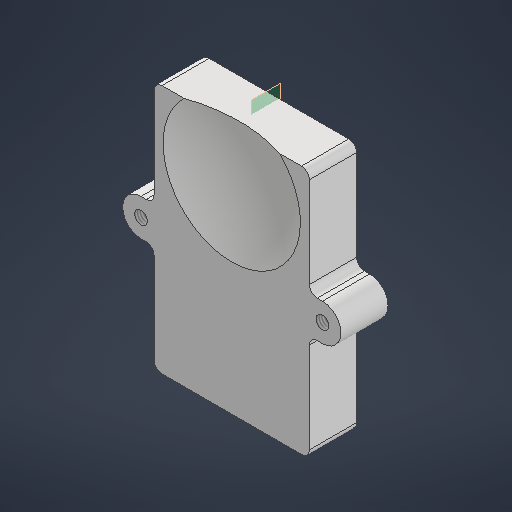
# Autodesk Inventor part: SphereMount
Saved by Autodesk Inventor 2025.1 (Build 291241020, 241B)
## iProperties
Created: 2024-09-20
Part Number: SphereMount
Material: Generic
Document SubType Name: Modeling
Designer: Sora
Density: 1 g/cm^3
Appearance: Default
Author: Sora
Autodesk Inventor part; units mm, degrees
ref_plane "YZ Plane" through (0, 0, 0) normal (1, 0, 0) x (0, 1, 0)
ref_plane "XZ Plane" through (0, 0, 0) normal (0, 1, 0) x (-1, 0, 0)
ref_plane "XY Plane" through (0, 0, 0) normal (0, 0, 1) x (1, 0, 0)
sketch "Sketch1" plane through (0, 0, 0) normal (0, 0, 1) x (1, 0, 0)
  arc A0 (-3.85, 3.05) -> (-3.85, -3.95) centre (-3.85, -0.45) ccw projected
  arc A1 (-1.4191, -5) -> (-2.85, -3.95) centre (-2.85, -5.45) ccw projected
  line L0 (-2.85, -3.95) -> (-3.85, -3.95) projected
  arc A2 (-1.35, -5.45) -> (-1.4191, -5) centre (-2.85, -5.45) ccw projected
  line L1 (-1.35, -5.45) -> (-1.35, -6) projected
  line L2 (-1.35, -6) -> (-1.35, -14.05) projected
  line L3 (-1.35, -14.05) -> (-1.35, -15.05) projected
  line L4 (-1.35, -15.05) -> (-1.35, -22.75) projected
  arc A3 (-1.35, -22.75) -> (0.15, -24.25) centre (0.15, -22.75) ccw projected
  line L5 (0.15, -24.25) -> (2.6, -24.25) projected
  line L6 (24.3, -24.25) -> (2.6, -24.25) projected
  line L7 (24.3, -24.25) -> (26.75, -24.25) projected
  arc A4 (26.75, -24.25) -> (28.25, -22.75) centre (26.75, -22.75) ccw projected
  line L8 (28.25, -22.75) -> (28.25, -15.05) projected
  line L9 (28.25, -15.05) -> (28.25, -14.05) projected
  line L10 (28.25, -14.05) -> (28.25, -6) projected
  line L11 (28.25, -6) -> (28.25, -5.45) projected
  arc A5 (28.3191, -5) -> (28.25, -5.45) centre (29.75, -5.45) ccw projected
  arc A6 (29.75, -3.95) -> (28.3191, -5) centre (29.75, -5.45) ccw projected
  arc A7 (30.75, -3.95) -> (30.75, 3.05) centre (30.75, -0.45) ccw projected
  line L12 (30.75, -3.95) -> (29.75, -3.95) projected
  line L13 (29.75, 3.05) -> (30.75, 3.05) projected
  arc A8 (28.25, 4.55) -> (29.75, 3.05) centre (29.75, 4.55) ccw projected
  line L14 (28.25, 4.55) -> (28.25, 5) projected
  line L15 (28.25, 5) -> (28.25, 6) projected
  line L16 (28.25, 6) -> (28.25, 21.85) projected
  arc A9 (28.25, 21.85) -> (26.75, 23.35) centre (26.75, 21.85) ccw projected
  line L17 (25.45, 23.35) -> (26.55, 23.35) projected
  line L18 (26.75, 23.35) -> (26.55, 23.35) projected
  line L19 (0.35, 23.35) -> (0.15, 23.35) projected
  arc A10 (0.15, 23.35) -> (-1.35, 21.85) centre (0.15, 21.85) ccw projected
  line L20 (0.35, 23.35) -> (1.45, 23.35) projected
  line L21 (-1.35, 5) -> (-1.35, 21.15) projected
  line L22 (-1.35, 21.85) -> (-1.35, 21.15) projected
  line L23 (-1.35, 5) -> (-1.35, 4.55) projected
  arc A11 (-2.85, 3.05) -> (-1.35, 4.55) centre (-2.85, 4.55) ccw projected
  line L24 (-3.85, 3.05) -> (-2.85, 3.05) projected
  line L25 (1.45, 23.35) -> (25.45, 23.35)
  point P0 (0, 0)
  constraints: 2 end point, 1 horizontal
extrude "Extrusion1" add sketch "Sketch1" along normal blind 9
ref_plane "Work Plane1" through (13.45, 4.55, 0) normal (-1, 0, 0) x (0, 0, 1)
sketch "Sketch2" plane through (13.45, 4.55, 0) normal (-1, 0, 0) x (0, 0, 1)
  line L0 (9, -8.5) -> (9, -1.5) projected
  circle A0 centre (36, 9.4) radius 30
  line L1 (9, 9.4) -> (36, 9.4)
  line L2 (36, 9.4) -> (66, 9.4)
  line L3 (9, 9.4) -> (6, 9.4)
  line L4 (-3, 9.8) -> (-3, 9) projected
  line L5 (9, -1.5) -> (9, -8.5) projected
  line L6 (9, -8.5) -> (9, -10) projected
  line L7 (9, -10) -> (9, -27.3) projected
  line L8 (9, -27.3) -> (9, -28.8) projected
  line L9 (9, -28.8) -> (9, -27.3) projected
  line L10 (9, -27.3) -> (9, -10) projected
  line L11 (9, -10) -> (9, -8.5) projected
  line L12 (9, -8.5) -> (9, -1.5) projected
  line L13 (9, -1.5) -> (9, 0) projected
  line L14 (9, 0) -> (9, 17.3) projected
  line L15 (9, 17.3) -> (9, 18.8) projected
  line L16 (9, 18.8) -> (9, 17.3) projected
  line L17 (9, 17.3) -> (9, 0) projected
  line L18 (9, 0) -> (9, -1.5) projected
  line L19 (9, 9.4) -> (-3, 9.4)
  point P0 (0, -4.55)
  dimension "d2" = 60
  dimension "d3" = 27
  constraints: 8 end point, 4 horizontal, 2 point on circle, 1 centre point, 1 midpoint, 1 point on line
  measures "d2" diameter of A0
  measures "d3" distance of L1.start L1.end
revolve "Revolution1" cut sketch "Sketch2" angle 360 about axis through (13.45, 13.95, 9) along (0, 0, 1) contours A0 L3 L14 L13 L0 | L0 L13 L14 L1 L2 A0
shell "Shell1" thickness 1 removed faces 1 at (9.0167, -11.7167, 0)
sketch "Sketch4" plane through (26.75, 22.35, 8) normal (0, 0, -1) x (-1, 0, 0)
  arc A0 (2.983, 0) -> (23.617, 0) centre (13.3, -8.4) ccw projected
  arc A1 (30.6, -25.3) -> (30.6, -20.3) centre (30.6, -22.8) ccw projected
  line L0 (29.6, -20.3) -> (30.6, -20.3) projected
  arc A2 (27.1, -17.8) -> (29.6, -20.3) centre (29.6, -17.8) ccw projected
  line L1 (27.1, -0.5) -> (27.1, -17.8) projected
  arc A3 (27.1, -0.5) -> (26.6, 0) centre (26.6, -0.5) ccw projected
  line L2 (23.617, 0) -> (26.6, 0) projected
  arc A4 (0, 0) -> (-0.5, -0.5) centre (0, -0.5) ccw projected
  line L3 (-0.5, -17.8) -> (-0.5, -0.5) projected
  arc A5 (-3, -20.3) -> (-0.5, -17.8) centre (-3, -17.8) ccw projected
  line L4 (-4, -20.3) -> (-3, -20.3) projected
  arc A6 (-4, -20.3) -> (-4, -25.3) centre (-4, -22.8) ccw projected
  line L5 (-3, -25.3) -> (-4, -25.3) projected
  arc A7 (-0.5, -27.8) -> (-3, -25.3) centre (-3, -27.8) ccw projected
  line L6 (-0.5, -45.1) -> (-0.5, -27.8) projected
  arc A8 (-0.5, -45.1) -> (0, -45.6) centre (0, -45.1) ccw projected
  line L7 (26.6, -45.6) -> (0, -45.6) projected
  arc A9 (26.6, -45.6) -> (27.1, -45.1) centre (26.6, -45.1) ccw projected
  line L8 (27.1, -27.8) -> (27.1, -45.1) projected
  arc A10 (29.6, -25.3) -> (27.1, -27.8) centre (29.6, -27.8) ccw projected
  line L9 (30.6, -25.3) -> (29.6, -25.3) projected
  line L10 (-0.5, -27.8) -> (-0.5, -17.8)
  line L11 (27.1, -27.8) -> (27.1, -17.8)
  line L12 (0, 0) -> (2.983, 0) projected
  point P0 (26.75, -22.35)
  constraints: 4 end point, 3 tangent, 1 collinear, 1 parallel
extrude "Extrusion2" add sketch "Sketch4" along normal up to surface (8 mm away) contours L10 A7 L5 A6 L4 A5 | A2 L0 A1 L9 A10 L11
sketch "Sketch5" plane through (0, 0, 0) normal (0, 0, -1) x (-1, 0, 0)
  circle A0 centre (-30.75, -0.45) radius 1.7 projected
  circle A1 centre (3.85, -0.45) radius 1.7 projected
  point P0 (0, 0)
hole "Hole1" at (30.75, -0.45, 0) at (-3.85, -0.45, 0) direction (0, 0, 1) diameter 2.459 end through all thread size "M3x0.5" class "6H" standard "ANSI Metric M Profile"
sketch "Sketch6" plane through (0.15, -24.25, 0) normal (0, -1, 0) x (1, 0, 0)
  line L0 (0, 0) -> (26.6, 0) projected
  line L1 (26.6, 0) -> (26.6, 9) projected
  line L2 (0, 9) -> (26.6, 9) projected
  line L3 (0, 0) -> (0, 9) projected
  line L4 (2.45, -3) -> (2.45, 0) projected
  line L5 (24.15, -3) -> (24.15, 0) projected
  line L6 (2.45, 0) -> (24.15, 0)
  line L7 (24.15, 0) -> (24.15, 7)
  line L8 (24.15, 7) -> (2.45, 7)
  line L9 (2.45, 7) -> (2.45, 0)
  point P0 (-0.15, 0)
  dimension "d15" = 2
  constraints: 8 end point, 2 parallel, 1 collinear, 1 horizontal, 1 perpendicular
  measures "d15" distance between parallel lines of L2 L8
extrude "Extrusion3" cut sketch "Sketch6" against normal blind 9 contours L9 L8 L7 L0
body "Solid1"
